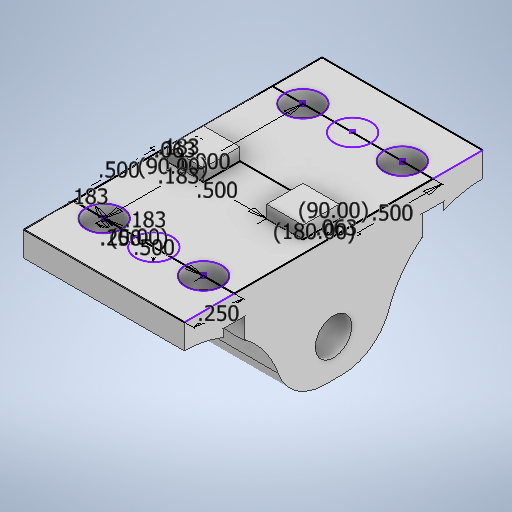
# Autodesk Inventor part: Odom Connector v2
Saved by Autodesk Inventor 2025.1 (Build 291241020, 241B)
## iProperties
Created: 2025-01-14
Part Number: Odom Connector v2
Material: Generic
Document SubType Name: Modeling
Designer: AtuStem
Density: 1 g/cm^3
Appearance: Default
Author: AtuStem
Autodesk Inventor part; units mm, degrees
ref_plane "YZ Plane" through (0, 0, 0) normal (1, 0, 0) x (0, 1, 0)
ref_plane "XZ Plane" through (0, 0, 0) normal (0, 1, 0) x (-1, 0, 0)
ref_plane "XY Plane" through (0, 0, 0) normal (0, 0, 1) x (1, 0, 0)
sketch "Sketch4" plane through (0, 0, 0) normal (0, 1, 0) x (-1, 0, 0)
  line L0 (0, 0) -> (4.6482, 0)
  line L1 (4.6482, 0) -> (4.6482, 4.6482)
  line L2 (4.6482, 4.6482) -> (0, 4.6482)
  line L3 (0, 4.6482) -> (0, 0)
  line L4 (4.6482, 0) -> (-10.1321, 0)
  line L5 (-8.0518, 4.6482) -> (-12.7, 4.6482)
  line L6 (-8.0518, 0) -> (-8.0518, 4.6482)
  line L7 (-12.7, 4.6482) -> (-12.7, 0)
  line L8 (-12.7, 0) -> (-8.0518, 0)
  line L9 (4.6482, 2.3241) -> (6.2357, 2.3241)
  line L10 (6.2357, 2.3241) -> (6.2357, 15.0241)
  line L11 (-12.7, 2.3241) -> (-14.2875, 2.3241)
  line L12 (-12.7, 2.3241) -> (-11.1125, 2.3241) construction
  line L13 (-14.2875, 2.3241) -> (-14.2875, -10.3759)
  line L14 (6.2357, 15.0241) -> (-14.2875, 15.0241)
  line L15 (-14.2875, 15.0241) -> (-14.2875, -10.3759)
  line L16 (-14.2875, -10.3759) -> (6.2357, -10.3759)
  line L17 (6.2357, -10.3759) -> (6.2357, 15.0241)
  line L18 (6.2357, 15.0241) -> (-14.2875, 15.0241)
  line L19 (-14.2875, 15.0241) -> (-14.2875, 21.3741)
  line L20 (-14.2875, 21.3741) -> (6.2357, 21.3741)
  line L21 (6.2357, 21.3741) -> (6.2357, 15.0241)
  line L22 (-14.2875, -10.3759) -> (-14.2875, -16.7259)
  line L23 (-14.2875, -16.7259) -> (6.2357, -16.7259)
  line L24 (6.2357, -16.7259) -> (6.2357, -10.3759)
  circle A0 centre (-4.0259, 15.0241) radius 2.3241
  circle A1 centre (-4.0259, -10.3759) radius 2.3241
  line L25 (-4.0259, 15.0241) -> (2.3241, 15.0241)
  line L26 (-4.0259, 15.0241) -> (2.3241, 15.0241) construction
  circle A2 centre (2.3241, 15.0241) radius 2.3241
  circle A3 centre (-10.3759, 15.0241) radius 2.3241
  circle A4 centre (2.3241, -10.3759) radius 2.3241
  circle A5 centre (-10.3759, -10.3759) radius 2.3241
  dimension "d46" = 4.6482
  dimension "d47" = 4.6482
  dimension "d50" = 12.7
  dimension "d59" = 1.5875
  dimension "d60" = 12.7
  dimension "d61" = 90
  dimension "d62" = 1.5875
  dimension "d63" = 180
  dimension "d64" = 12.7
  dimension "d65" = 90
  dimension "d66" = 6.35
  dimension "d67" = 4.6482
  dimension "d90" = 6.35
  dimension "d91" = 0
  dimension "d92" = 4.6482
  dimension "d95" = 12.7
  dimension "d98" = 25.4
  constraints: 54 end point, 10 horizontal, 6 centre point, 6 parallel, 5 perpendicular, 4 symmetric about line, 3 collinear, 3 midpoint, 1 coincident, 1 vertical, 15 other
  measures "d46" distance of L2.end L1.end
  measures "d47" distance of L1.end L0.end
  measures "d50" distance of L1.end L5.start
  measures "d59" distance of L9.start L9.end
  measures "d60" distance of L9.end L10.end
  measures "d61" angle of L10 L9
  measures "d62" distance of L11.start L11.end
  measures "d63" angle of L11 L12
  measures "d64" distance of L11.end L13.end
  measures "d65" angle of L13 L11
  measures "d66" distance of L18.end L19.end
  measures "d67" diameter of A0
  measures "d90" distance of L25.start L25.end
  measures "d91" distance between parallel lines of L25 L26
  measures "d92" diameter of A2
  measures "d95" distance of A2.centre A3.centre
  measures "d98" distance of A2.centre A4.centre
extrude "Extrusion4" add sketch "Sketch4" along normal blind 1.5875 contours L3 L2 L1 L0 | L4 L8 L7 L5 L6
extrude "Extrusion5" add sketch "Sketch4" against normal blind 15.875
sketch "Sketch5" plane through (0, -15.875, 0) normal (0, -1, 0) x (1, 0, 0)
  circle A0 centre (4.0259, 15.0241) radius 2.3241 projected
  circle A1 centre (4.0259, 15.0241) radius 2.3241
  circle A2 centre (4.0259, -10.3759) radius 2.3241 projected
  circle A3 centre (4.0259, -10.3759) radius 2.3241
  line L0 (4.0259, 15.0241) -> (10.3759, 15.0241)
  circle A4 centre (10.3759, 15.0241) radius 2.3241
  line L1 (10.3759, 15.0241) -> (10.3759, 8.6741)
  circle A5 centre (-2.3241, 15.0241) radius 2.3241
  circle A6 centre (10.3759, -10.3759) radius 2.3241
  circle A7 centre (-2.3241, -10.3759) radius 2.3241
  point P0 (0, 0)
  dimension "d101" = 6.35
  dimension "d102" = 4.6482
  dimension "d103" = 6.35
  dimension "d106" = 12.7
  dimension "d109" = 25.4
  constraints: 6 centre point, 4 end point, 3 coincident, 2 horizontal, 2 vertical, 6 other
  measures "d101" distance of L0.start L0.end
  measures "d102" diameter of A4
  measures "d103" distance of L1.start L1.end
  measures "d106" distance of L1.start A5.centre
  measures "d109" distance of L1.start A6.centre
sketch "Sketch6" plane through (-6.2357, 0, -16.7259) normal (-1, 0, 0) x (0, 0, 1)
  line L0 (38.1, 0) -> (0, 0) projected
  line L1 (38.1, 0) -> (0, 0)
  line L2 (0, 0) -> (19.05, 0)
  line L3 (19.05, 0) -> (19.05, -11.1125)
  circle A0 centre (19.05, -11.1125) radius 2.3241
  point P0 (16.7259, 0)
  dimension "d81" = 11.1125
  dimension "d82" = 4.6482
  constraints: 6 end point, 1 centre point, 1 coincident, 1 collinear, 1 midpoint, 1 perpendicular
  measures "d81" distance of L2.end L3.end
  measures "d82" diameter of A0
hole "Hole4" at (-6.2357, -11.1125, 2.3241) direction (1, 0, 0) diameter 4.6482 depth 32.3342 tip angle 118 counterbore diameter 8.255 counterbore depth 3.175
hole "Hole5" at (10.3759, -15.875, 15.0241) at (-2.3241, -15.875, 15.0241) at (-2.3241, -15.875, -10.3759) at (10.3759, -15.875, -10.3759) direction (0, 1, 0) diameter 4.6482 depth 32.3342 tip angle 118 counterbore diameter 8.255 counterbore depth 12.7
fillet "Fillet5" radius 12.7 2 edges at (4.0259, -15.875, 21.3741) (4.0259, -15.875, -16.7259) inverted yes
fillet "Fillet6" radius 6.35 2 edges at (4.0259, -15.875, 8.6741) (4.0259, -15.875, -4.0259)
body "Solid2"
